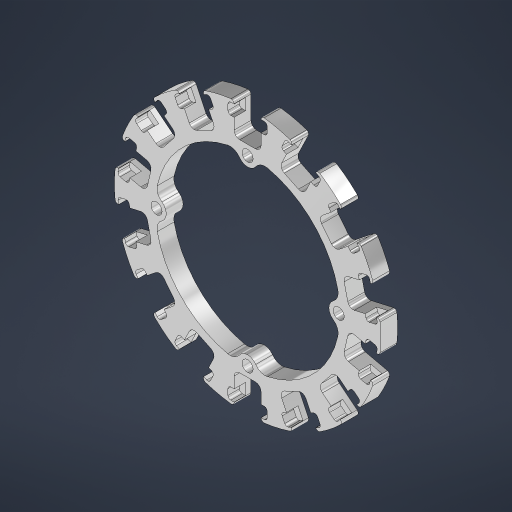
# Autodesk Inventor part: Wheel_Flame
Saved by Autodesk Inventor 2024.2 (Build 282272000, 272)
## iProperties
Created: 2023-12-20
Part Number: Wheel_Flame
Material: 一般
Document SubType Name: Modeling
Designer: Hanaoka
Density: 1 g/cm^3
Appearance: クロム - つや出し
Author: Hanaoka
Autodesk Inventor part; units mm, degrees
ref_plane "YZ Plane" through (0, 0, 0) normal (1, 0, 0) x (0, 1, 0)
ref_plane "XZ Plane" through (0, 0, 0) normal (0, 1, 0) x (-1, 0, 0)
ref_plane "XY Plane" through (0, 0, 0) normal (0, 0, 1) x (1, 0, 0)
sketch "スケッチ1" plane through (0, 0, 0) normal (0, 0, 1) x (1, 0, 0)
  circle A0 centre (0, 0) radius 25 construction
  line L0 (-2.4, 24.8845) -> (-2.4, 19)
  line L1 (-1.4, 18) -> (1.4, 18)
  line L2 (2.4, 19) -> (2.4, 24.8845)
  line L3 (0, 25) -> (0, 18) construction
  line L4 (-2.4, 23.025) -> (-3, 23.025)
  line L5 (-3.5, 22.525) -> (-3.5, 21.475)
  line L6 (-3, 20.975) -> (-2.4, 20.975)
  line L7 (2.4, 23.025) -> (3, 23.025)
  line L8 (3.5, 22.525) -> (3.5, 21.475)
  line L9 (3, 20.975) -> (2.4, 20.975)
  arc A1 (-3, 23.025) -> (-3.5, 22.525) centre (-3, 22.525) ccw
  arc A2 (-3.5, 21.475) -> (-3, 20.975) centre (-3, 21.475) ccw
  arc A3 (3.5, 22.525) -> (3, 23.025) centre (3, 22.525) ccw
  arc A4 (3, 20.975) -> (3.5, 21.475) centre (3, 21.475) ccw
  arc A5 (-2.4, 19) -> (-1.4, 18) centre (-1.4, 19) ccw
  arc A6 (1.4, 18) -> (2.4, 19) centre (1.4, 19) ccw
  arc A7 (-10.4061, 16.0771) -> (-9.0713, 15.61) centre (-9.5051, 16.511) ccw
  arc A8 (-6.5486, 16.8249) -> (-6.0815, 18.1597) centre (-6.9824, 17.7258) ccw
  line L10 (-9.0713, 15.61) -> (-6.5486, 16.8249)
  line L11 (-6.3978, 20.1995) -> (-6.9384, 19.9391)
  arc A9 (-6.3978, 20.1995) -> (-6.1643, 20.8669) centre (-6.6147, 20.65) ccw
  line L12 (-6.6198, 21.8129) -> (-6.1643, 20.8669)
  arc A10 (-6.6198, 21.8129) -> (-7.2873, 22.0465) centre (-7.0703, 21.596) ccw
  line L13 (-7.8278, 21.7861) -> (-7.2873, 22.0465)
  line L14 (-11.8036, 17.5962) -> (-11.263, 17.8565)
  line L15 (-6.0815, 18.1597) -> (-8.6347, 23.4615)
  line L16 (-10.8471, 22.5242) -> (-7.8099, 16.2174) construction
  line L17 (-12.9593, 21.3789) -> (-10.4061, 16.0771)
  arc A11 (-12.471, 17.8297) -> (-11.8036, 17.5962) centre (-12.0206, 18.0467) ccw
  line L18 (-12.1525, 19.7035) -> (-12.6931, 19.4432)
  line L19 (-12.9266, 18.7757) -> (-12.471, 17.8297)
  arc A12 (-12.6931, 19.4432) -> (-12.9266, 18.7757) centre (-12.4761, 18.9927) ccw
  arc A13 (-16.3512, 9.9699) -> (-14.9459, 10.1283) centre (-15.7277, 10.7517) ccw
  arc A14 (-13.2001, 12.3174) -> (-13.3584, 13.7227) centre (-13.9819, 12.9409) ccw
  line L20 (-14.9459, 10.1283) -> (-13.2001, 12.3174)
  line L21 (-14.5284, 15.4232) -> (-14.9025, 14.9541)
  arc A15 (-14.5284, 15.4232) -> (-14.6076, 16.1259) centre (-14.9194, 15.7349) ccw
  line L22 (-15.4285, 16.7805) -> (-14.6076, 16.1259)
  arc A16 (-15.4285, 16.7805) -> (-16.1312, 16.7013) centre (-15.7403, 16.3896) ccw
  line L23 (-16.5053, 16.2322) -> (-16.1312, 16.7013)
  line L24 (-18.2694, 10.7322) -> (-17.8953, 11.2013)
  line L25 (-13.3584, 13.7227) -> (-17.9591, 17.3916)
  line L26 (-19.5458, 15.5872) -> (-14.073, 11.2228) construction
  line L27 (-20.9519, 13.6389) -> (-16.3512, 9.9699)
  arc A17 (-18.972, 10.653) -> (-18.2694, 10.7322) centre (-18.6603, 11.0439) ccw
  line L28 (-19.498, 12.4795) -> (-19.8721, 12.0104)
  line L29 (-19.793, 11.3077) -> (-18.972, 10.653)
  arc A18 (-19.8721, 12.0104) -> (-19.793, 11.3077) centre (-19.4812, 11.6986) ccw
  arc A19 (-19.0577, 1.8881) -> (-17.8602, 2.6405) centre (-18.8352, 2.863) ccw
  arc A20 (-17.2372, 5.3703) -> (-17.9896, 6.5677) centre (-18.2121, 5.5928) ccw
  line L30 (-17.8602, 2.6405) -> (-17.2372, 5.3703)
  line L31 (-19.7816, 7.5922) -> (-19.9151, 7.0072)
  arc A21 (-19.7816, 7.5922) -> (-20.1578, 8.1909) centre (-20.269, 7.7034) ccw
  line L32 (-21.1814, 8.4245) -> (-20.1578, 8.1909)
  arc A22 (-21.1814, 8.4245) -> (-21.7802, 8.0483) centre (-21.2927, 7.9371) ccw
  line L33 (-21.9137, 7.4634) -> (-21.7802, 8.0483)
  line L34 (-21.1167, 1.7426) -> (-20.9832, 2.3275)
  line L35 (-17.9896, 6.5677) -> (-23.7266, 7.8772)
  line L36 (-24.3732, 5.563) -> (-17.5487, 4.0054) construction
  line L37 (-24.7947, 3.1975) -> (-19.0577, 1.8881)
  arc A23 (-21.7154, 1.3664) -> (-21.1167, 1.7426) centre (-21.6041, 1.8539) ccw
  line L38 (-22.9818, 2.7837) -> (-23.1153, 2.1988)
  line L39 (-22.7391, 1.6) -> (-21.7154, 1.3664)
  arc A24 (-23.1153, 2.1988) -> (-22.7391, 1.6) centre (-22.6278, 2.0875) ccw
  arc A25 (-17.9896, -6.5677) -> (-17.2372, -5.3703) centre (-18.2121, -5.5928) ccw
  arc A26 (-17.8602, -2.6405) -> (-19.0577, -1.8881) centre (-18.8352, -2.863) ccw
  line L40 (-17.2372, -5.3703) -> (-17.8602, -2.6405)
  line L41 (-21.1167, -1.7426) -> (-20.9832, -2.3275)
  arc A27 (-21.1167, -1.7426) -> (-21.7154, -1.3664) centre (-21.6041, -1.8539) ccw
  line L42 (-22.7391, -1.6) -> (-21.7154, -1.3664)
  arc A28 (-22.7391, -1.6) -> (-23.1153, -2.1988) centre (-22.6278, -2.0875) ccw
  line L43 (-22.9818, -2.7837) -> (-23.1153, -2.1988)
  line L44 (-19.7816, -7.5922) -> (-19.9151, -7.0072)
  line L45 (-19.0577, -1.8881) -> (-24.7947, -3.1975)
  line L46 (-24.3732, -5.563) -> (-17.5487, -4.0054) construction
  line L47 (-23.7266, -7.8772) -> (-17.9896, -6.5677)
  arc A29 (-20.1578, -8.1909) -> (-19.7816, -7.5922) centre (-20.269, -7.7034) ccw
  line L48 (-21.9137, -7.4634) -> (-21.7802, -8.0483)
  line L49 (-21.1814, -8.4245) -> (-20.1578, -8.1909)
  arc A30 (-21.7802, -8.0483) -> (-21.1814, -8.4245) centre (-21.2927, -7.9371) ccw
  arc A31 (-13.3584, -13.7227) -> (-13.2001, -12.3174) centre (-13.9819, -12.9409) ccw
  arc A32 (-14.9459, -10.1283) -> (-16.3512, -9.9699) centre (-15.7277, -10.7517) ccw
  line L50 (-13.2001, -12.3174) -> (-14.9459, -10.1283)
  line L51 (-18.2694, -10.7322) -> (-17.8953, -11.2013)
  arc A33 (-18.2694, -10.7322) -> (-18.972, -10.653) centre (-18.6603, -11.0439) ccw
  line L52 (-19.793, -11.3077) -> (-18.972, -10.653)
  arc A34 (-19.793, -11.3077) -> (-19.8721, -12.0104) centre (-19.4812, -11.6986) ccw
  line L53 (-19.498, -12.4795) -> (-19.8721, -12.0104)
  line L54 (-14.5284, -15.4232) -> (-14.9025, -14.9541)
  line L55 (-16.3512, -9.9699) -> (-20.9519, -13.6389)
  line L56 (-19.5458, -15.5872) -> (-14.073, -11.2228) construction
  line L57 (-17.9591, -17.3916) -> (-13.3584, -13.7227)
  arc A35 (-14.6076, -16.1259) -> (-14.5284, -15.4232) centre (-14.9194, -15.7349) ccw
  line L58 (-16.5053, -16.2322) -> (-16.1312, -16.7013)
  line L59 (-15.4285, -16.7805) -> (-14.6076, -16.1259)
  arc A36 (-16.1312, -16.7013) -> (-15.4285, -16.7805) centre (-15.7403, -16.3896) ccw
  arc A37 (-6.0815, -18.1597) -> (-6.5486, -16.8249) centre (-6.9824, -17.7258) ccw
  arc A38 (-9.0713, -15.61) -> (-10.4061, -16.0771) centre (-9.5051, -16.511) ccw
  line L60 (-6.5486, -16.8249) -> (-9.0713, -15.61)
  line L61 (-11.8036, -17.5962) -> (-11.263, -17.8565)
  arc A39 (-11.8036, -17.5962) -> (-12.471, -17.8297) centre (-12.0206, -18.0467) ccw
  line L62 (-12.9266, -18.7757) -> (-12.471, -17.8297)
  arc A40 (-12.9266, -18.7757) -> (-12.6931, -19.4432) centre (-12.4761, -18.9927) ccw
  line L63 (-12.1525, -19.7035) -> (-12.6931, -19.4432)
  line L64 (-6.3978, -20.1995) -> (-6.9384, -19.9391)
  line L65 (-10.4061, -16.0771) -> (-12.9593, -21.3789)
  line L66 (-10.8471, -22.5242) -> (-7.8099, -16.2174) construction
  line L67 (-8.6347, -23.4615) -> (-6.0815, -18.1597)
  arc A41 (-6.1643, -20.8669) -> (-6.3978, -20.1995) centre (-6.6147, -20.65) ccw
  line L68 (-7.8278, -21.7861) -> (-7.2873, -22.0465)
  line L69 (-6.6198, -21.8129) -> (-6.1643, -20.8669)
  arc A42 (-7.2873, -22.0465) -> (-6.6198, -21.8129) centre (-7.0703, -21.596) ccw
  arc A43 (2.4, -19) -> (1.4, -18) centre (1.4, -19) ccw
  arc A44 (-1.4, -18) -> (-2.4, -19) centre (-1.4, -19) ccw
  line L70 (1.4, -18) -> (-1.4, -18)
  line L71 (-3, -20.975) -> (-2.4, -20.975)
  arc A45 (-3, -20.975) -> (-3.5, -21.475) centre (-3, -21.475) ccw
  line L72 (-3.5, -22.525) -> (-3.5, -21.475)
  arc A46 (-3.5, -22.525) -> (-3, -23.025) centre (-3, -22.525) ccw
  line L73 (-2.4, -23.025) -> (-3, -23.025)
  line L74 (3, -20.975) -> (2.4, -20.975)
  line L75 (-2.4, -19) -> (-2.4, -24.8845)
  line L76 (0, -25) -> (0, -18) construction
  line L77 (2.4, -24.8845) -> (2.4, -19)
  arc A47 (3.5, -21.475) -> (3, -20.975) centre (3, -21.475) ccw
  line L78 (2.4, -23.025) -> (3, -23.025)
  line L79 (3.5, -22.525) -> (3.5, -21.475)
  arc A48 (3, -23.025) -> (3.5, -22.525) centre (3, -22.525) ccw
  arc A49 (10.4061, -16.0771) -> (9.0713, -15.61) centre (9.5051, -16.511) ccw
  arc A50 (6.5486, -16.8249) -> (6.0815, -18.1597) centre (6.9824, -17.7258) ccw
  line L80 (9.0713, -15.61) -> (6.5486, -16.8249)
  line L81 (6.3978, -20.1995) -> (6.9384, -19.9391)
  arc A51 (6.3978, -20.1995) -> (6.1643, -20.8669) centre (6.6147, -20.65) ccw
  line L82 (6.6198, -21.8129) -> (6.1643, -20.8669)
  arc A52 (6.6198, -21.8129) -> (7.2873, -22.0465) centre (7.0703, -21.596) ccw
  line L83 (7.8278, -21.7861) -> (7.2873, -22.0465)
  line L84 (11.8036, -17.5962) -> (11.263, -17.8565)
  line L85 (6.0815, -18.1597) -> (8.6347, -23.4615)
  line L86 (10.8471, -22.5242) -> (7.8099, -16.2174) construction
  line L87 (12.9593, -21.3789) -> (10.4061, -16.0771)
  arc A53 (12.471, -17.8297) -> (11.8036, -17.5962) centre (12.0206, -18.0467) ccw
  line L88 (12.1525, -19.7035) -> (12.6931, -19.4432)
  line L89 (12.9266, -18.7757) -> (12.471, -17.8297)
  arc A54 (12.6931, -19.4432) -> (12.9266, -18.7757) centre (12.4761, -18.9927) ccw
  arc A55 (16.3512, -9.9699) -> (14.9459, -10.1283) centre (15.7277, -10.7517) ccw
  arc A56 (13.2001, -12.3174) -> (13.3584, -13.7227) centre (13.9819, -12.9409) ccw
  line L90 (14.9459, -10.1283) -> (13.2001, -12.3174)
  line L91 (14.5284, -15.4232) -> (14.9025, -14.9541)
  arc A57 (14.5284, -15.4232) -> (14.6076, -16.1259) centre (14.9194, -15.7349) ccw
  line L92 (15.4285, -16.7805) -> (14.6076, -16.1259)
  arc A58 (15.4285, -16.7805) -> (16.1312, -16.7013) centre (15.7403, -16.3896) ccw
  line L93 (16.5053, -16.2322) -> (16.1312, -16.7013)
  line L94 (18.2694, -10.7322) -> (17.8953, -11.2013)
  line L95 (13.3584, -13.7227) -> (17.9591, -17.3916)
  line L96 (19.5458, -15.5872) -> (14.073, -11.2228) construction
  line L97 (20.9519, -13.6389) -> (16.3512, -9.9699)
  arc A59 (18.972, -10.653) -> (18.2694, -10.7322) centre (18.6603, -11.0439) ccw
  line L98 (19.498, -12.4795) -> (19.8721, -12.0104)
  line L99 (19.793, -11.3077) -> (18.972, -10.653)
  arc A60 (19.8721, -12.0104) -> (19.793, -11.3077) centre (19.4812, -11.6986) ccw
  arc A61 (19.0577, -1.8881) -> (17.8602, -2.6405) centre (18.8352, -2.863) ccw
  arc A62 (17.2372, -5.3703) -> (17.9896, -6.5677) centre (18.2121, -5.5928) ccw
  line L100 (17.8602, -2.6405) -> (17.2372, -5.3703)
  line L101 (19.7816, -7.5922) -> (19.9151, -7.0072)
  arc A63 (19.7816, -7.5922) -> (20.1578, -8.1909) centre (20.269, -7.7034) ccw
  line L102 (21.1814, -8.4245) -> (20.1578, -8.1909)
  arc A64 (21.1814, -8.4245) -> (21.7802, -8.0483) centre (21.2927, -7.9371) ccw
  line L103 (21.9137, -7.4634) -> (21.7802, -8.0483)
  line L104 (21.1167, -1.7426) -> (20.9832, -2.3275)
  line L105 (17.9896, -6.5677) -> (23.7266, -7.8772)
  line L106 (24.3732, -5.563) -> (17.5487, -4.0054) construction
  line L107 (24.7947, -3.1975) -> (19.0577, -1.8881)
  arc A65 (21.7154, -1.3664) -> (21.1167, -1.7426) centre (21.6041, -1.8539) ccw
  line L108 (22.9818, -2.7837) -> (23.1153, -2.1988)
  line L109 (22.7391, -1.6) -> (21.7154, -1.3664)
  arc A66 (23.1153, -2.1988) -> (22.7391, -1.6) centre (22.6278, -2.0875) ccw
  arc A67 (17.9896, 6.5677) -> (17.2372, 5.3703) centre (18.2121, 5.5928) ccw
  arc A68 (17.8602, 2.6405) -> (19.0577, 1.8881) centre (18.8352, 2.863) ccw
  line L110 (17.2372, 5.3703) -> (17.8602, 2.6405)
  line L111 (21.1167, 1.7426) -> (20.9832, 2.3275)
  arc A69 (21.1167, 1.7426) -> (21.7154, 1.3664) centre (21.6041, 1.8539) ccw
  line L112 (22.7391, 1.6) -> (21.7154, 1.3664)
  arc A70 (22.7391, 1.6) -> (23.1153, 2.1988) centre (22.6278, 2.0875) ccw
  line L113 (22.9818, 2.7837) -> (23.1153, 2.1988)
  line L114 (19.7816, 7.5922) -> (19.9151, 7.0072)
  line L115 (19.0577, 1.8881) -> (24.7947, 3.1975)
  line L116 (24.3732, 5.563) -> (17.5487, 4.0054) construction
  line L117 (23.7266, 7.8772) -> (17.9896, 6.5677)
  arc A71 (20.1578, 8.1909) -> (19.7816, 7.5922) centre (20.269, 7.7034) ccw
  line L118 (21.9137, 7.4634) -> (21.7802, 8.0483)
  line L119 (21.1814, 8.4245) -> (20.1578, 8.1909)
  arc A72 (21.7802, 8.0483) -> (21.1814, 8.4245) centre (21.2927, 7.9371) ccw
  arc A73 (13.3584, 13.7227) -> (13.2001, 12.3174) centre (13.9819, 12.9409) ccw
  arc A74 (14.9459, 10.1283) -> (16.3512, 9.9699) centre (15.7277, 10.7517) ccw
  line L120 (13.2001, 12.3174) -> (14.9459, 10.1283)
  line L121 (18.2694, 10.7322) -> (17.8953, 11.2013)
  arc A75 (18.2694, 10.7322) -> (18.972, 10.653) centre (18.6603, 11.0439) ccw
  line L122 (19.793, 11.3077) -> (18.972, 10.653)
  arc A76 (19.793, 11.3077) -> (19.8721, 12.0104) centre (19.4812, 11.6986) ccw
  line L123 (19.498, 12.4795) -> (19.8721, 12.0104)
  line L124 (14.5284, 15.4232) -> (14.9025, 14.9541)
  line L125 (16.3512, 9.9699) -> (20.9519, 13.6389)
  line L126 (19.5458, 15.5872) -> (14.073, 11.2228) construction
  line L127 (17.9591, 17.3916) -> (13.3584, 13.7227)
  arc A77 (14.6076, 16.1259) -> (14.5284, 15.4232) centre (14.9194, 15.7349) ccw
  line L128 (16.5053, 16.2322) -> (16.1312, 16.7013)
  line L129 (15.4285, 16.7805) -> (14.6076, 16.1259)
  arc A78 (16.1312, 16.7013) -> (15.4285, 16.7805) centre (15.7403, 16.3896) ccw
  arc A79 (6.0815, 18.1597) -> (6.5486, 16.8249) centre (6.9824, 17.7258) ccw
  arc A80 (9.0713, 15.61) -> (10.4061, 16.0771) centre (9.5051, 16.511) ccw
  line L130 (6.5486, 16.8249) -> (9.0713, 15.61)
  line L131 (11.8036, 17.5962) -> (11.263, 17.8565)
  arc A81 (11.8036, 17.5962) -> (12.471, 17.8297) centre (12.0206, 18.0467) ccw
  line L132 (12.9266, 18.7757) -> (12.471, 17.8297)
  arc A82 (12.9266, 18.7757) -> (12.6931, 19.4432) centre (12.4761, 18.9927) ccw
  line L133 (12.1525, 19.7035) -> (12.6931, 19.4432)
  line L134 (6.3978, 20.1995) -> (6.9384, 19.9391)
  line L135 (10.4061, 16.0771) -> (12.9593, 21.3789)
  line L136 (10.8471, 22.5242) -> (7.8099, 16.2174) construction
  line L137 (8.6347, 23.4615) -> (6.0815, 18.1597)
  arc A83 (6.1643, 20.8669) -> (6.3978, 20.1995) centre (6.6147, 20.65) ccw
  line L138 (7.8278, 21.7861) -> (7.2873, 22.0465)
  line L139 (6.6198, 21.8129) -> (6.1643, 20.8669)
  arc A84 (7.2873, 22.0465) -> (6.6198, 21.8129) centre (7.0703, 21.596) ccw
  circle A85 centre (0, 0) radius 23.75
  circle A86 centre (0, 0) radius 16.5
  circle A87 centre (0, 0) radius 2
  line L140 (-2, -3.5) -> (2, -3.5)
  line L141 (3.5, -2) -> (3.5, 2)
  line L142 (2, 3.5) -> (-2, 3.5)
  line L143 (-3.5, 2) -> (-3.5, -2)
  line L144 (-3.5, -3.5) -> (3.5, 3.5) construction
  line L145 (3.5, -3.5) -> (-3.5, 3.5) construction
  arc A88 (-2, 3.5) -> (-3.5, 2) centre (-2, 2) ccw
  arc A89 (-3.5, -2) -> (-2, -3.5) centre (-2, -2) ccw
  arc A90 (2, -3.5) -> (3.5, -2) centre (2, -2) ccw
  arc A91 (3.5, 2) -> (2, 3.5) centre (2, 2) ccw
  line L146 (-1.75, 16.4069) -> (-1.75, 3.5)
  line L147 (1.75, 3.5) -> (1.75, 16.4069)
  circle A92 centre (0, 16.25) radius 1
  line L148 (0, -35) -> (0, 35) projected
  circle A93 centre (0, 16.25) radius 1.75
  circle A94 centre (-16.25, 0) radius 1
  line L149 (-3.5, 1.75) -> (-16.4069, 1.75)
  line L150 (-16.4069, -1.75) -> (-3.5, -1.75)
  circle A95 centre (0, -16.25) radius 1
  line L151 (-1.75, -3.5) -> (-1.75, -16.4069)
  line L152 (1.75, -16.4069) -> (1.75, -3.5)
  circle A96 centre (16.25, 0) radius 1
  line L153 (3.5, -1.75) -> (16.4069, -1.75)
  line L154 (16.4069, 1.75) -> (3.5, 1.75)
  circle A97 centre (-16.25, 0) radius 1.75
  circle A98 centre (0, -16.25) radius 1.75
  circle A99 centre (16.25, 0) radius 1.75
  line L155 (-1.3229, 1.5) -> (1.3229, 1.5)
  circle A100 centre (0, 0) radius 14.5
  point P0 (-2.4, 18)
  point P1 (2.4, 18)
  point P2 (3.5, 23.025)
  point P3 (3.5, 20.975)
  point P4 (-3.5, 22)
  point P5 (-9.9722, 15.1761)
  point P6 (-5.6476, 17.2588)
  point P7 (-5.9473, 20.4164)
  point P8 (-6.8368, 22.2634)
  point P9 (-12.6988, 18.3027)
  point P10 (-15.5693, 9.3464)
  point P11 (-12.5766, 13.0992)
  point P12 (-14.2167, 15.8141)
  point P13 (-15.8195, 17.0923)
  point P14 (-19.3825, 10.9804)
  point P15 (-18.0828, 1.6655)
  point P16 (-17.0147, 6.3452)
  point P17 (-19.6703, 8.0796)
  point P18 (-21.6689, 8.5358)
  point P19 (-22.2272, 1.4832)
  point P20 (-17.0147, -6.3452)
  point P21 (-18.0828, -1.6655)
  point P22 (-21.2279, -1.2551)
  point P23 (-23.2265, -1.7113)
  point P24 (-20.6696, -8.3077)
  point P25 (-12.5766, -13.0992)
  point P26 (-15.5693, -9.3464)
  point P27 (-18.5811, -10.3413)
  point P28 (-20.1839, -11.6194)
  point P29 (-15.0181, -16.4532)
  point P30 (-5.6476, -17.2588)
  point P31 (-9.9722, -15.1761)
  point P32 (-12.2541, -17.3792)
  point P33 (-13.1436, -19.2262)
  point P34 (-6.3921, -21.3399)
  point P35 (2.4, -18)
  point P36 (-2.4, -18)
  point P37 (-3.5, -20.975)
  point P38 (-3.5, -23.025)
  point P39 (3.5, -22)
  point P40 (9.9722, -15.1761)
  point P41 (5.6476, -17.2588)
  point P42 (5.9473, -20.4164)
  point P43 (6.8368, -22.2634)
  point P44 (12.6988, -18.3027)
  point P45 (15.5693, -9.3464)
  point P46 (12.5766, -13.0992)
  point P47 (14.2167, -15.8141)
  point P48 (15.8195, -17.0923)
  point P49 (19.3825, -10.9804)
  point P50 (18.0828, -1.6655)
  point P51 (17.0147, -6.3452)
  point P52 (19.6703, -8.0796)
  point P53 (21.6689, -8.5358)
  point P54 (22.2272, -1.4832)
  point P55 (17.0147, 6.3452)
  point P56 (18.0828, 1.6655)
  point P57 (21.2279, 1.2551)
  point P58 (23.2265, 1.7113)
  point P59 (20.6696, 8.3077)
  point P60 (12.5766, 13.0992)
  point P61 (15.5693, 9.3464)
  point P62 (18.5811, 10.3413)
  point P63 (20.1839, 11.6194)
  point P64 (15.0181, 16.4532)
  point P65 (5.6476, 17.2588)
  point P66 (9.9722, 15.1761)
  point P67 (12.2541, 17.3792)
  point P68 (13.1436, 19.2262)
  point P69 (6.3921, 21.3399)
  point P70 (-2.4, 23.6284)
  point P71 (-8.0897, 22.3298)
  point P72 (-12.4143, 20.2472)
  point P73 (-16.9771, 16.6085)
  point P74 (-19.9698, 12.8557)
  point P75 (-22.502, 7.5976)
  point P76 (-23.5701, 2.918)
  point P77 (-23.5701, -2.918)
  point P78 (-22.502, -7.5976)
  point P79 (-19.9698, -12.8557)
  point P80 (-16.9771, -16.6085)
  point P81 (-12.4143, -20.2472)
  point P82 (-8.0897, -22.3298)
  point P83 (-2.4, -23.6284)
  point P84 (2.4, -23.6284)
  point P85 (8.0897, -22.3298)
  point P86 (12.4143, -20.2472)
  point P87 (16.9771, -16.6085)
  point P88 (19.9698, -12.8557)
  point P89 (22.502, -7.5976)
  point P90 (23.5701, -2.918)
  point P91 (23.5701, 2.918)
  point P92 (22.502, 7.5976)
  point P93 (19.9698, 12.8557)
  point P94 (16.9771, 16.6085)
  point P95 (12.4143, 20.2472)
  point P96 (8.0897, 22.3298)
  point P97 (2.4, 23.6284)
  point P98 (1.75, 16.25)
  point P99 (16.4069, 1.75)
  point P100 (16.25, 1.75)
  point P101 (16.25, -1.75)
  point P102 (16.4069, -1.75)
  point P103 (1.75, -16.4069)
  point P104 (1.75, -16.25)
  point P105 (-1.75, -16.25)
  point P106 (-1.75, -16.4069)
  point P107 (-16.4069, -1.75)
  point P108 (-16.25, -1.75)
  point P109 (-16.25, 1.75)
  point P110 (-16.4069, 1.75)
  point P111 (-1.75, 16.25)
  point P112 (1.75, 14.394)
  point P113 (14.394, 1.75)
  point P114 (14.394, -1.75)
  point P115 (1.75, -14.394)
  point P116 (-1.75, -14.394)
  point P117 (-14.394, -1.75)
  point P118 (-14.394, 1.75)
  point P119 (-1.75, 14.394)
  point P120 (0, -14.5)
  point P121 (14.5, 0)
  point P122 (-14.5, 0)
  point P123 (0, 14.5)
  dimension "d14" = 47.5
  dimension "d0" = 50
  dimension "d1" = 4.8
  dimension "d2" = 0.5
  dimension "d5" = 2.05
  dimension "d7" = 1
  dimension "d8" = 7
  dimension "d9" = 3
  dimension "d12" = 360
  dimension "d19" = 33
  dimension "d20" = 4
  dimension "d21" = 1.5
  dimension "d22" = 4
  dimension "d23" = 3.5
  dimension "d24" = 2
  dimension "d25" = 3.5
  dimension "d28" = 360
  dimension "d32" = 360
  dimension "d35" = 1.5
  dimension "d38" = 6
  constraints: 310 end point, 235 point on line, 183 point on circle, 100 centre point, 22 tangent, 7 equal radius, 6 coincident, 6 perpendicular, 5 parallel, 4 equal length, 4 midpoint, 3 horizontal, 1 vertical, 703 other
  measures "d0" diameter of A0
  measures "d1" distance of point (-2.4, 18) point (2.4, 18)
  measures "d2" radius of A1
  measures "d5" distance between parallel lines of L6 L4
  measures "d7" radius of A5
  measures "d8" distance of L3.start L3.end
  measures "d9" vertical distance of point (-3.5, 22) L3.start
  measures "d19" diameter of A86
  measures "d20" diameter of A87
  measures "d21" radius of A88
  measures "d22" distance of L142.start L142.end
  measures "d23" distance between parallel lines of L147 L146
  measures "d24" diameter of A92
  measures "d25" diameter of A93
  measures "d35" distance from line of A0.centre L155
  measures "d38" distance of A3.centre A1.centre
extrude "押し出し1" add sketch "スケッチ1" along normal blind 2.05 contours L4 A1 L5 A2 L6 L0 A5 L1 A93 A86 A97 A98 L70 A44 L75 L71 A45 L72 A46 L73 A85 L67 L68 A42 L69 A41 L64 A37 L60 A38 L65 L61 A39 L62 A40 L63 L57 L58 A36 L59 A35 L54 A31 L50 A32 L55 L51 A33 L52 A34 L53 L47 L48 A30 L49 A29 L44 A25 L40 A26 L45 L41 A27 L42 A28 L43 L37 L38 A24 L39 A23 L34 A19 L30 A20 L35 L31 A21 L32 A22 L33 L27 L28 A18 L29 A17 L24 A13 L20 A14 L25 L21 A15 L22 A16 L23 L17 L18 A12 L19 A11 L14 A7 L10 A8 L15 L11 A9 L12 A10 L13 | A85 L137 L138 A84 L139 A83 L134 A79 L130 A80 L135 L131 A81 L132 A82 L133 L127 L128 A78 L129 A77 L124 A73 L120 A74 L125 L121 A75 L122 A76 L123 L117 L118 A72 L119 A71 L114 A67 L110 A68 L115 L111 A69 L112 A70 L113 L107 L108 A66 L109 A65 L104 A61 L100 A62 L105 L101 A63 L102 A64 L103 L97 L98 A60 L99 A59 L94 A55 L90 A56 L95 L91 A57 L92 A58 L93 L87 L88 A54 L89 A53 L84 A49 L80 A50 L85 L81 A51 L82 A52 L83 L77 L78 A48 L79 A47 L74 A43 L70 A98 A86 A99 A93 L1 A6 L2 L9 A4 L8 A3 L7 | A93 A86 A92 L148 | L148 A92 A86 A93 | A93 L148 A92 A86 | A86 L147 A93 | A93 L146 A86 | A86 A92 L148 A93 | A86 A99 L154 | L149 A97 A86 | A99 A86 A96 | A86 A96 A99 | A97 A86 A94 | A86 A94 A97 | A97 L150 A86 | A86 L153 A99 | L151 A98 A86 | A86 A98 L152 | A98 A86 A95 L148 | L148 A95 A86 A98 | A86 A95 L148 A98 | A98 L148 A95 A86
extrude "押し出し2" add sketch "スケッチ1" against normal blind 0.95 contours L4 A1 L5 A2 L6 L0 A5 L1 A93 A86 A97 A98 L70 A44 L75 L71 A45 L72 A46 L73 A85 L67 L68 A42 L69 A41 L64 A37 L60 A38 L65 L61 A39 L62 A40 L63 L57 L58 A36 L59 A35 L54 A31 L50 A32 L55 L51 A33 L52 A34 L53 L47 L48 A30 L49 A29 L44 A25 L40 A26 L45 L41 A27 L42 A28 L43 L37 L38 A24 L39 A23 L34 A19 L30 A20 L35 L31 A21 L32 A22 L33 L27 L28 A18 L29 A17 L24 A13 L20 A14 L25 L21 A15 L22 A16 L23 L17 L18 A12 L19 A11 L14 A7 L10 A8 L15 L11 A9 L12 A10 L13 | L0 L6 A2 L5 A1 L4 | A85 L137 L138 A84 L139 A83 L134 A79 L130 A80 L135 L131 A81 L132 A82 L133 L127 L128 A78 L129 A77 L124 A73 L120 A74 L125 L121 A75 L122 A76 L123 L117 L118 A72 L119 A71 L114 A67 L110 A68 L115 L111 A69 L112 A70 L113 L107 L108 A66 L109 A65 L104 A61 L100 A62 L105 L101 A63 L102 A64 L103 L97 L98 A60 L99 A59 L94 A55 L90 A56 L95 L91 A57 L92 A58 L93 L87 L88 A54 L89 A53 L84 A49 L80 A50 L85 L81 A51 L82 A52 L83 L77 L78 A48 L79 A47 L74 A43 L70 A98 A86 A99 A93 L1 A6 L2 L9 A4 L8 A3 L7 | A93 A86 A92 L148 | L148 A92 A86 A93 | L13 A10 L12 A9 L11 L15 | L7 A3 L8 A4 L9 L2 | A93 L148 A92 A86 | A86 L147 A93 | A93 L146 A86 | A86 A92 L148 A93 | L17 L14 A11 L19 A12 L18 | L137 L134 A83 L139 A84 L138 | L23 A16 L22 A15 L21 L25 | L133 A82 L132 A81 L131 L135 | A86 A99 L154 | L149 A97 A86 | L27 L24 A17 L29 A18 L28 | L127 L124 A77 L129 A78 L128 | A99 A86 A96 | A86 A96 A99 | A97 A86 A94 | A86 A94 A97 | L33 A22 L32 A21 L31 L35 | L123 A76 L122 A75 L121 L125 | A97 L150 A86 | L37 L34 A23 L39 A24 L38 | L117 L114 A71 L119 A72 L118 | A86 L153 A99 | L43 A28 L42 A27 L41 L45 | L113 A70 L112 A69 L111 L115 | L151 A98 A86 | L47 L44 A29 L49 A30 L48 | A86 A98 L152 | A98 A86 A95 L148 | L148 A95 A86 A98 | A86 A95 L148 A98 | L53 A34 L52 A33 L51 L55 | L107 L104 A65 L109 A66 L108 | A98 L148 A95 A86 | L57 L54 A35 L59 A36 L58 | L103 A64 L102 A63 L101 L105 | L63 A40 L62 A39 L61 L65 | L97 L94 A59 L99 A60 L98 | L67 L64 A41 L69 A42 L68 | L93 A58 L92 A57 L91 L95 | L74 A47 L79 A48 L78 L77 | L75 L73 A46 L72 A45 L71 | L87 L84 A53 L89 A54 L88 | L83 A52 L82 A51 L81 L85
fillet "フィレット2" radius 0.5 28 edges at (-2.4, 23.6284, 0.55) (-8.0897, 22.3298, 0.55) (-12.4143, 20.2472, 0.55) (-16.9771, 16.6085, 0.55) (-19.9698, 12.8557, 0.55) (-22.502, 7.5976, 0.55) (-23.5701, 2.918, 0.55) (-23.5701, -2.918, 0.55) (-22.502, -7.5976, 0.55) (-19.9698, -12.8557, 0.55) (-16.9771, -16.6085, 0.55) (-12.4143, -20.2472, 0.55) (-8.0897, -22.3298, 0.55) (-2.4, -23.6284, 0.55) (2.4, -23.6284, 0.55) (8.0897, -22.3298, 0.55) (12.4143, -20.2472, 0.55) (16.9771, -16.6085, 0.55) (22.502, -7.5976, 0.55) (23.5701, -2.918, 0.55) (23.5701, 2.918, 0.55) (22.502, 7.5976, 0.55) (19.9698, 12.8557, 0.55) (16.9771, 16.6085, 0.55) (12.4143, 20.2472, 0.55) (8.0897, 22.3298, 0.55) (2.4, 23.6284, 0.55) (19.9698, -12.8557, 0.55)
fillet "フィレット3" radius 2 8 edges at (-1.75, 16.4069, 0.55) (1.75, 16.4069, 0.55) (-16.4069, 1.75, 0.55) (-16.4069, -1.75, 0.55) (-1.75, -16.4069, 0.55) (1.75, -16.4069, 0.55) (16.4069, 1.75, 0.55) (16.4069, -1.75, 0.55)
